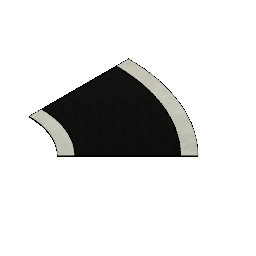
_Small Turn - Ruby.a3587e5a-fc20-4334-9f9f-3d097e04c7a0 (Autodesk Fusion 360 design; units mm, degrees)
Autodesk Fusion 360 part; units mm, degrees
sketch "Sketch1" plane through (0, 0, 0) normal (0, 0, 1) x (1, 0, 0)
  circle A0 centre (0, 0) radius 660.4
  circle A1 centre (0, 0) radius 1270
  line L0 (0, 0) -> (0, 1270)
  line L1 (0, 0) -> (1270, 0)
  line L2 (0, 0) -> (898.0256, 898.0256)
  line L3 (0, 0) -> (1270, 0) construction
  dimension "d1" = 1320.8
  dimension "d2" = 609.6
  dimension "d3" = 45
  constraint coincident A0.centre A1.centre
  constraint coincident A1 L0.end
  constraint vertical L0
  constraint coincident A1 L1.end
  constraint perpendicular L0 L1
  constraint horizontal L3
  measures "d1" diameter of A0
  measures "d3" angle of L2 L3
extrude "Extrude1" add sketch "Sketch1" along normal blind 6.35 contours A0 A1 L0 L2 makes body 1
sketch "Sketch2" plane through (0, 0, 6.35) normal (0, 0, 1) x (-1, 0, 0)
  line L0 (-466.9733, -466.9733) -> (-898.0256, -898.0256)
  arc A0 (-898.0256, -898.0256) -> (0, -1270) centre (0, 0) ccw
  line L1 (0, -1270) -> (0, -660.4)
  arc A1 (-466.9733, -466.9733) -> (0, -660.4) centre (0, 0) ccw
  line L2 (101.6, -1367.8319) -> (101.6, -549.486)
  arc A2 (-460.3873, -316.7032) -> (101.6, -549.486) centre (0, 0) ccw
  line L3 (-460.3873, -316.7032) -> (-1039.0452, -895.3611)
  arc A3 (-1039.0452, -895.3611) -> (101.6, -1367.8319) centre (0, 0) ccw
  line L4 (101.6, -549.486) -> (0, -549.486)
  line L5 (0, -549.486) -> (0, -1371.5989)
  line L6 (0, -1371.5989) -> (101.6, -1371.5989)
  line L7 (101.6, -1371.5989) -> (101.6, -549.486)
  line L8 (-466.9733, -466.9733) -> (-395.1313, -395.1313)
  line L9 (-898.0256, -898.0256) -> (-969.8677, -969.8677)
  dimension "d6" = -101.6
  dimension "d7" = 101.6
  constraint horizontal L4
  constraint vertical L5
  constraint horizontal L6
  constraint vertical L7
  constraint coincident L0.start A1.start
  constraint coincident A2 L8.end
  constraint parallel L0 L8
  constraint coincident L0.end A0.start
  constraint coincident A3 L9.end
  constraint parallel L0 L9
  measures "d7" distance of L2.end L4.end
extrude "Extrude1'" add sketch "Sketch2" against normal blind 6.35 separate body contours A1 A2 L5 L8 | A0 A3 L5 L6 L9 makes body 2 at (53.0458, 623.0565, 6.35) makes body 3 at (232.4048, 1314.7857, 6.35) in component "45"
copy_body "CutPasteBodies1" bodies 1 removing the originals makes body 4 in component "45"
component "45" placed x (1, 0, 0) y (0, 1, 0) z (0, 0, 1) at (0, 0, 0)
